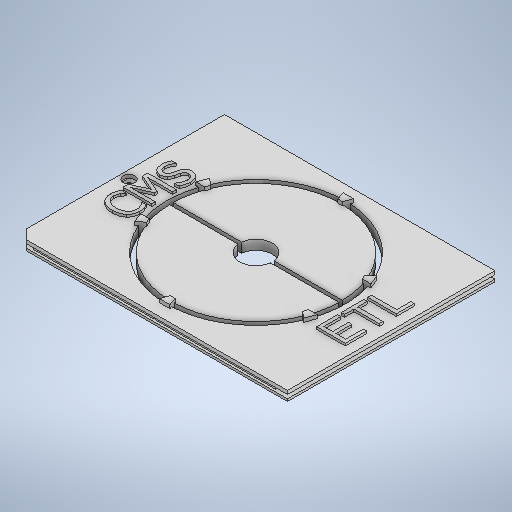
# Autodesk Inventor part: Tamale Souvenir
Saved by Autodesk Inventor 2025 (Build 290162000, 162)
## iProperties
Created: 2025-02-25
Part Number: Tamale Souvenir
Material: Generic
Document SubType Name: Modeling
Designer: Caleb Fangmeier
Density: 1 g/cm^3
Appearance: Default
Author: Caleb Fangmeier
Autodesk Inventor part; units mm, degrees
ref_plane "YZ Plane" through (0, 0, 0) normal (1, 0, 0) x (0, 1, 0)
ref_plane "XZ Plane" through (0, 0, 0) normal (0, 1, 0) x (-1, 0, 0)
ref_plane "XY Plane" through (0, 0, 0) normal (0, 0, 1) x (1, 0, 0)
sketch "Sketch1" plane through (0, 0, 0) normal (0, 1, 0) x (-1, 0, 0)
  line L0 (-28.75, -22.05) -> (28.75, -22.05)
  line L1 (28.75, -22.05) -> (28.75, 22.05)
  line L2 (28.75, 22.05) -> (-28.75, 22.05)
  line L3 (-28.75, 22.05) -> (-28.75, -22.05)
  line L4 (-28.75, -22.05) -> (28.75, 22.05) construction
  line L5 (28.75, -22.05) -> (-28.75, 22.05) construction
  point P0 (0, 0)
  dimension "d0" = 44.1
  dimension "d1" = 57.5
  constraints: 12 end point, 2 midpoint, 2 parallel, 1 horizontal, 1 perpendicular
  measures "d0" distance of L0.end L1.end
  measures "d1" distance of L1.end L2.end
extrude "Extrusion1" add sketch "Sketch1" along normal blind 0.5
sketch "Sketch2" plane through (0, 0.5, 0) normal (0, 1, 0) x (1, 0, 0)
  line L0 (-28.75, 22.05) -> (-28.75, -22.05) projected
  line L1 (-28.75, -22.05) -> (28.75, -22.05) projected
  line L2 (-28.75, -20.05) -> (-26.75, -22.05)
  point P0 (0, 0)
  dimension "d4" = 45
  dimension "d5" = 2
  constraints: 2 end point, 2 point on line
  measures "d4" angle of L2 L0
  measures "d5" distance of L2.start L0.end
extrude "Extrusion2" cut sketch "Sketch2" against normal through all
sketch "Sketch3" plane through (0, 0.5, 0) normal (0, 1, 0) x (1, 0, 0)
  line L0 (25.75, 21.55) -> (-25.75, 21.55)
  line L1 (-25.75, 21.55) -> (-25.75, -21.55)
  line L2 (-25.75, -21.55) -> (25.75, -21.55)
  line L3 (25.75, -21.55) -> (25.75, 21.55)
  line L4 (25.75, 21.55) -> (-25.75, -21.55) construction
  line L5 (-25.75, 21.55) -> (25.75, -21.55) construction
  line L6 (-26.75, -22.05) -> (28.75, -22.05) projected
  line L7 (-28.75, 22.05) -> (-28.75, -20.05) projected
  point P0 (0, 0)
  dimension "d8" = 0.5
  dimension "d9" = 3
  constraints: 12 end point, 2 midpoint, 2 parallel, 1 horizontal, 1 perpendicular
  measures "d8" distance between parallel lines of L6 L2
  measures "d9" distance between parallel lines of L7 L1
extrude "Extrusion3" add sketch "Sketch3" along normal blind 0.8
sketch "Sketch4" plane through (0, 1.3, 0) normal (0, 1, 0) x (1, 0, 0)
  line L0 (-25.75, 21.55) -> (-25.75, -21.55) projected
  line L1 (25.75, 0.25) -> (-25.75, 0.25)
  line L2 (-25.75, 0.25) -> (-25.75, -0.25)
  line L3 (-25.75, -0.25) -> (25.75, -0.25)
  line L4 (25.75, -0.25) -> (25.75, 0.25)
  line L5 (25.75, 0.25) -> (-25.75, -0.25) construction
  line L6 (-25.75, 0.25) -> (25.75, -0.25) construction
  line L7 (25.75, 21.55) -> (-25.75, 21.55) projected
  line L8 (0.25, -21.55) -> (-0.25, -21.55)
  line L9 (-0.25, -21.55) -> (-0.25, 21.55)
  line L10 (-0.25, 21.55) -> (0.25, 21.55)
  line L11 (0.25, 21.55) -> (0.25, -21.55)
  line L12 (0.25, -21.55) -> (-0.25, 21.55) construction
  line L13 (-0.25, -21.55) -> (0.25, 21.55) construction
  point P0 (0, 0)
  point P1 (0.25, -0.25)
  point P2 (0.25, 0.25)
  point P3 (-0.25, 0.25)
  point P4 (-0.25, -0.25)
  dimension "d12" = 0.5
  dimension "d13" = 0.5
  constraints: 24 end point, 4 midpoint, 4 parallel, 2 horizontal, 2 perpendicular, 2 point on line
  measures "d12" distance between parallel lines of L9 L11
  measures "d13" distance between parallel lines of L3 L1
extrude "Extrusion4" cut sketch "Sketch4" against normal up to surface (0.8 mm away) contours L1 L9 L3 L0 | L7 L11 L1 L9 | L1 L11 L3 L9 | L3 L11 L8 L9 | L1 L4 L3 L11
sketch "Sketch5" plane through (0, 1.3, 0) normal (0, 1, 0) x (1, 0, 0)
  line L0 (28.75, 22.05) -> (-28.75, 22.05)
  line L1 (-28.75, 22.05) -> (-28.75, -22.05)
  line L2 (-28.75, -22.05) -> (28.75, -22.05)
  line L3 (28.75, -22.05) -> (28.75, 22.05)
  line L4 (28.75, 22.05) -> (-28.75, -22.05) construction
  line L5 (-28.75, 22.05) -> (28.75, -22.05) construction
  point P0 (0, 0)
  constraints: 12 end point, 2 midpoint, 2 parallel, 1 coincident, 1 horizontal, 1 perpendicular
extrude "Extrusion5" add sketch "Sketch5" along normal blind 0.75
sketch "Sketch6" plane through (0, 2.05, 0) normal (0, 1, 0) x (1, 0, 0)
  line L0 (-28.75, 22.05) -> (-28.75, -22.05) projected
  line L1 (-28.75, -22.05) -> (28.75, -22.05) projected
  line L2 (-26.75, -22.05) -> (-28.75, -20.05) projected
  line L3 (-28.75, -20.05) -> (-26.75, -22.05)
  point P0 (0, 0)
  constraints: 2 end point, 1 collinear
extrude "Extrusion6" cut sketch "Sketch6" against normal through all
sketch "Sketch7" plane through (0, 2.05, 0) normal (0, 1, 0) x (1, 0, 0)
  circle A0 centre (0, 0) radius 19
  circle A1 centre (0, 0) radius 20
  dimension "d20" = 38
  dimension "d21" = 40
  constraints: 2 centre point, 2 coincident
  measures "d20" diameter of A0
  measures "d21" diameter of A1
extrude "Extrusion7" add sketch "Sketch7" against normal up to surface (2.05 mm away)
extrude "Extrusion8" cut sketch "Sketch7" against normal through all contours A0
sketch "Sketch8" plane through (0, 2.05, 0) normal (0, 1, 0) x (1, 0, 0)
  circle A0 centre (0, 0) radius 18
  circle A1 centre (0, 0) radius 19 projected
  dimension "d26" = 1
  constraints: 1 centre point, 1 coincident
  measures "d26" radial gap between concentric circles of A1 A0
extrude "Extrusion9" add sketch "Sketch8" against normal up to surface (2.05 mm away) contours A0
sketch "Sketch9" plane through (0, 2.05, 0) normal (0, 1, 0) x (1, 0, 0)
  line L0 (18.25, 0.375) -> (-18.25, 0.375)
  line L1 (-18.25, 0.375) -> (-18.25, -0.375)
  line L2 (-18.25, -0.375) -> (18.25, -0.375)
  line L3 (18.25, -0.375) -> (18.25, 0.375)
  line L4 (18.25, 0.375) -> (-18.25, -0.375) construction
  line L5 (-18.25, 0.375) -> (18.25, -0.375) construction
  point P0 (0, 0)
  dimension "d29" = 0.75
  dimension "d30" = 36.5
  constraints: 12 end point, 2 midpoint, 2 parallel, 1 horizontal, 1 perpendicular
  measures "d29" distance of L0.end L1.end
  measures "d30" distance of L0.start L0.end
extrude "Extrusion10" cut sketch "Sketch9" against normal blind 10
sketch "Sketch10" plane through (0, 2.05, 0) normal (0, 1, 0) x (1, 0, 0)
  line L0 (-16.4621, -6.804) -> (-16.8041, -5.8643)
  line L1 (-16.8041, -5.8643) -> (-18.6315, -5.8643)
  line L2 (-18.6315, -5.8643) -> (-17.8619, -7.9786)
  line L3 (-17.8619, -7.9786) -> (-16.4621, -6.804)
  line L4 (17.9961, -0.375) -> (-17.9961, -0.375) projected
  circle A0 centre (0, 0) radius 19 projected
  line L5 (0.608, -17.8024) -> (-0.392, -17.7937)
  line L6 (-0.392, -17.7937) -> (-1.032, -19.5053)
  line L7 (-1.032, -19.5053) -> (1.218, -19.525)
  line L8 (1.218, -19.525) -> (0.608, -17.8024)
  line L9 (16.8879, -5.6651) -> (16.5296, -6.5986)
  line L10 (16.5296, -6.5986) -> (17.9087, -7.7975)
  line L11 (17.9087, -7.7975) -> (18.715, -5.697)
  line L12 (18.715, -5.697) -> (16.8879, -5.6651)
  line L13 (-18.266, 0) -> (18.3496, 0)
  line L14 (-16.4621, 6.804) -> (-16.8041, 5.8643)
  line L15 (-16.8041, 5.8643) -> (-18.6315, 5.8643)
  line L16 (-18.6315, 5.8643) -> (-17.8619, 7.9786)
  line L17 (-17.8619, 7.9786) -> (-16.4621, 6.804)
  line L18 (0.608, 17.8024) -> (-0.392, 17.7937)
  line L19 (-0.392, 17.7937) -> (-1.032, 19.5053)
  line L20 (-1.032, 19.5053) -> (1.218, 19.525)
  line L21 (1.218, 19.525) -> (0.608, 17.8024)
  line L22 (16.8879, 5.6651) -> (16.5296, 6.5986)
  line L23 (16.5296, 6.5986) -> (17.9087, 7.7975)
  line L24 (17.9087, 7.7975) -> (18.715, 5.697)
  line L25 (18.715, 5.697) -> (16.8879, 5.6651)
  dimension "d33" = 1
  dimension "d34" = 2.25
  dimension "d35" = 110
  dimension "d36" = 110
  dimension "d37" = 110
  dimension "d41" = 139
  constraints: 50 end point, 12 symmetric about line, 1 horizontal, 1 parallel, 17 other
  measures "d33" distance of L0.start L0.end
  measures "d34" distance of L1.end L2.end
  measures "d35" angle of L0 L1
  measures "d36" angle of L3 L0
  measures "d37" angle of L4 L2
extrude "Extrusion11" add sketch "Sketch10" along normal blind 0.75 and the other way blind 2.05 contours L3 A0 L1 L0 | L3 L2 L1 A0 | L6 L5 L8 A0 | A0 L8 L7 L6 | L15 L16 L17 A0 | A0 L17 L14 L15 | L10 L9 L12 A0 | A0 L12 L11 L10 | L19 L20 L21 A0 | A0 L21 L18 L19 | L23 L24 L25 A0 | A0 L25 L22 L23
sketch "Sketch11" plane through (0, 2.05, 0) normal (0, 1, 0) x (1, 0, 0)
  circle A0 centre (0, 0) radius 3.4726
  constraints: 1 centre point, 1 coincident
extrude "Extrusion12" cut sketch "Sketch11" against normal through all
sketch "Sketch12" plane through (0, 2.05, 0) normal (0, 1, 0) x (1, 0, 0)
  line L0 (-28.75, 22.05) -> (-28.75, -20.05) projected
  line L1 (20.6121, -8.4043) -> (20.6121, 11.3007) construction
  line L2 (20.6121, 11.3007) -> (27.7105, 11.3007) construction
  line L3 (27.7105, 11.3007) -> (27.7105, -8.4043) construction
  line L4 (27.7105, -8.4043) -> (20.6121, -8.4043) construction
  line L5 (-25.7514, -8.2683) -> (-25.7514, -0.1864) construction
  line L6 (-25.7514, -0.1864) -> (-22.5947, -0.1864) construction
  line L7 (-22.5947, -0.1864) -> (-22.5947, -8.2683) construction
  line L8 (-22.5947, -8.2683) -> (-25.7514, -8.2683) construction
  spline S0 degree 2 poles (-19.4339, -5.2678) (-19.4339, -5.861) (-19.8343, -6.8644) (-20.2347, -7.2302) knots 0 0 0 1 2 2 2
  spline S1 degree 2 poles (-20.2347, -7.2302) (-20.6302, -7.596) (-21.8166, -7.9964) (-22.5877, -7.9964) knots 0 0 0 1 2 2 2
  spline S2 degree 2 poles (-22.5877, -7.9964) (-23.3539, -7.9964) (-24.4909, -7.6059) (-24.911, -7.2352) knots 0 0 0 1 2 2 2
  spline S3 degree 2 poles (-24.911, -7.2352) (-25.3213, -6.8694) (-25.7514, -5.8708) (-25.7514, -5.2529) knots 0 0 0 1 2 2 2
  spline S4 degree 2 poles (-25.7514, -5.2529) (-25.7514, -4.9464) (-25.6624, -4.4076) (-25.5932, -4.1802) knots 0 0 0 1 2 2 2
  spline S5 degree 2 poles (-25.5932, -4.1802) (-25.529, -3.9825) (-25.3461, -3.5722) (-25.2373, -3.3695) knots 0 0 0 1 2 2 2
  line L9 (-25.2373, -3.3695) -> (-24.2585, -3.3695)
  line L10 (-24.2585, -3.3695) -> (-24.2585, -3.4338)
  spline S6 degree 2 poles (-24.2585, -3.4338) (-24.3574, -3.5426) (-24.6342, -3.8787) (-24.7677, -4.1209) knots 0 0 0 1 2 2 2
  spline S7 degree 2 poles (-24.7677, -4.1209) (-24.8962, -4.3533) (-25.0593, -4.902) (-25.0593, -5.2579) knots 0 0 0 1 2 2 2
  spline S8 degree 2 poles (-25.0593, -5.2579) (-25.0593, -5.6484) (-24.738, -6.3454) (-24.4315, -6.6074) knots 0 0 0 1 2 2 2
  spline S9 degree 2 poles (-24.4315, -6.6074) (-24.1201, -6.8644) (-23.176, -7.1511) (-22.5877, -7.1511) knots 0 0 0 1 2 2 2
  spline S10 degree 2 poles (-22.5877, -7.1511) (-21.9599, -7.1511) (-21.0553, -6.8496) (-20.7439, -6.5876) knots 0 0 0 1 2 2 2
  spline S11 degree 2 poles (-20.7439, -6.5876) (-20.4423, -6.3306) (-20.1358, -5.6435) (-20.1358, -5.2579) knots 0 0 0 1 2 2 2
  spline S12 degree 2 poles (-20.1358, -5.2579) (-20.1358, -4.9069) (-20.3089, -4.3088) (-20.4374, -4.0764) knots 0 0 0 1 2 2 2
  spline S13 degree 2 poles (-20.4374, -4.0764) (-20.5659, -3.854) (-20.8328, -3.5228) (-20.9268, -3.4289) knots 0 0 0 1 2 2 2
  line L11 (-20.9268, -3.4289) -> (-20.9268, -3.3695)
  line L12 (-20.9268, -3.3695) -> (-19.9579, -3.3695)
  spline S14 degree 2 poles (-19.9579, -3.3695) (-19.864, -3.5722) (-19.6909, -3.9281) (-19.6119, -4.1802) knots 0 0 0 1 2 2 2
  spline S15 degree 2 poles (-19.6119, -4.1802) (-19.5229, -4.4472) (-19.4339, -4.902) (-19.4339, -5.2678) knots 0 0 0 1 2 2 2
  line L13 (-19.5427, 2.6168) -> (-19.5427, 1.8061)
  line L14 (-19.5427, 1.8061) -> (-24.7974, 1.8061)
  line L15 (-24.7974, 1.8061) -> (-21.2234, 0.2143)
  line L16 (-21.2234, 0.2143) -> (-21.2234, -0.28)
  line L17 (-21.2234, -0.28) -> (-24.7974, -1.8569)
  line L18 (-24.7974, -1.8569) -> (-19.5427, -1.8569)
  line L19 (-19.5427, -1.8569) -> (-19.5427, -2.6132)
  line L20 (-19.5427, -2.6132) -> (-25.6427, -2.6132)
  line L21 (-25.6427, -2.6132) -> (-25.6427, -1.5059)
  line L22 (-25.6427, -1.5059) -> (-22.2466, 0.0166)
  line L23 (-22.2466, 0.0166) -> (-25.6427, 1.4897)
  line L24 (-25.6427, 1.4897) -> (-25.6427, 2.6168)
  line L25 (-25.6427, 2.6168) -> (-19.5427, 2.6168)
  spline S16 degree 2 poles (-19.4339, 5.5531) (-19.4339, 4.8907) (-19.7107, 3.9613) (-19.9085, 3.551) knots 0 0 0 1 2 2 2
  line L26 (-19.9085, 3.551) -> (-20.9268, 3.551)
  line L27 (-20.9268, 3.551) -> (-20.9268, 3.6104)
  spline S17 degree 2 poles (-20.9268, 3.6104) (-20.5511, 4.0108) (-20.1358, 5.0241) (-20.1358, 5.4937) knots 0 0 0 1 2 2 2
  spline S18 degree 2 poles (-20.1358, 5.4937) (-20.1358, 6.166) (-20.6944, 6.8531) (-21.1542, 6.8531) knots 0 0 0 1 2 2 2
  spline S19 degree 2 poles (-21.1542, 6.8531) (-21.52, 6.8531) (-21.9747, 6.4923) (-22.0884, 6.1018) knots 0 0 0 1 2 2 2
  spline S20 degree 2 poles (-22.0884, 6.1018) (-22.1675, 5.82) (-22.2763, 5.3504) (-22.3653, 4.9994) knots 0 0 0 1 2 2 2
  spline S21 degree 2 poles (-22.3653, 4.9994) (-22.4493, 4.683) (-22.7014, 4.1838) (-22.9041, 3.991) knots 0 0 0 1 2 2 2
  spline S22 degree 2 poles (-22.9041, 3.991) (-23.1068, 3.8031) (-23.6505, 3.5955) (-24.0064, 3.5955) knots 0 0 0 1 2 2 2
  spline S23 degree 2 poles (-24.0064, 3.5955) (-24.7479, 3.5955) (-25.7514, 4.7523) (-25.7514, 5.647) knots 0 0 0 1 2 2 2
  spline S24 degree 2 poles (-25.7514, 5.647) (-25.7514, 6.1611) (-25.5487, 7.0706) (-25.3559, 7.4612) knots 0 0 0 1 2 2 2
  line L28 (-25.3559, 7.4612) -> (-24.3871, 7.4612)
  line L29 (-24.3871, 7.4612) -> (-24.3871, 7.4018)
  spline S25 degree 2 poles (-24.3871, 7.4018) (-24.654, 7.1102) (-25.0495, 6.2006) (-25.0495, 5.7014) knots 0 0 0 1 2 2 2
  spline S26 degree 2 poles (-25.0495, 5.7014) (-25.0495, 5.1378) (-24.5205, 4.4408) (-24.0905, 4.4408) knots 0 0 0 1 2 2 2
  spline S27 degree 2 poles (-24.0905, 4.4408) (-23.7049, 4.4408) (-23.2452, 4.8511) (-23.1414, 5.2367) knots 0 0 0 1 2 2 2
  spline S28 degree 2 poles (-23.1414, 5.2367) (-23.0721, 5.4937) (-22.8942, 6.2402) (-22.82, 6.4873) knots 0 0 0 1 2 2 2
  spline S29 degree 2 poles (-22.82, 6.4873) (-22.6273, 7.1151) (-21.8512, 7.6984) (-21.2827, 7.6984) knots 0 0 0 1 2 2 2
  spline S30 degree 2 poles (-21.2827, 7.6984) (-20.9218, 7.6984) (-20.2298, 7.4068) (-19.9875, 7.1448) knots 0 0 0 1 2 2 2
  spline S31 degree 2 poles (-19.9875, 7.1448) (-19.7206, 6.8531) (-19.4339, 6.1117) (-19.4339, 5.5531) knots 0 0 0 1 2 2 2
  line L30 (26.7121, -7.7302) -> (20.6121, -7.7302)
  line L31 (20.6121, -7.7302) -> (20.6121, -3.3132)
  line L32 (20.6121, -3.3132) -> (21.3328, -3.3132)
  line L33 (21.3328, -3.3132) -> (21.3328, -6.9212)
  line L34 (21.3328, -6.9212) -> (23.1972, -6.9212)
  line L35 (23.1972, -6.9212) -> (23.1972, -3.5411)
  line L36 (23.1972, -3.5411) -> (23.9179, -3.5411)
  line L37 (23.9179, -3.5411) -> (23.9179, -6.9212)
  line L38 (23.9179, -6.9212) -> (25.9915, -6.9212)
  line L39 (25.9915, -6.9212) -> (25.9915, -3.1738)
  line L40 (25.9915, -3.1738) -> (26.7121, -3.1738)
  line L41 (26.7121, -3.1738) -> (26.7121, -7.7302)
  line L42 (26.7121, -0.5097) -> (21.3328, -0.5097)
  line L43 (21.3328, -0.5097) -> (21.3328, -2.5182)
  line L44 (21.3328, -2.5182) -> (20.6121, -2.5182)
  line L45 (20.6121, -2.5182) -> (20.6121, 2.3172)
  line L46 (20.6121, 2.3172) -> (21.3328, 2.3172)
  line L47 (21.3328, 2.3172) -> (21.3328, 0.2993)
  line L48 (21.3328, 0.2993) -> (26.7121, 0.2993)
  line L49 (26.7121, 0.2993) -> (26.7121, -0.5097)
  line L50 (26.7121, 3.1122) -> (20.6121, 3.1122)
  line L51 (20.6121, 3.1122) -> (20.6121, 3.9212)
  line L52 (20.6121, 3.9212) -> (25.9915, 3.9212)
  line L53 (25.9915, 3.9212) -> (25.9915, 6.9247)
  line L54 (25.9915, 6.9247) -> (26.7121, 6.9247)
  line L55 (26.7121, 6.9247) -> (26.7121, 3.1122)
  point P0 (0, 0)
  constraints: 2 parallel, 4 other
emboss "Emboss1" sketch "Sketch12" operation add depth 0.5 direction (0, -1, 0)
sketch "Sketch13" plane through (0, 2.05, 0) normal (0, 1, 0) x (1, 0, 0)
  circle A0 centre (-26.9813, 0) radius 1.25
  point P0 (0, 0)
  dimension "d52" = 2.5
  constraints: 1 centre point
  measures "d52" diameter of A0
extrude "Extrusion13" cut sketch "Sketch13" against normal through all
equation "\"d36\" = d35"
body "Solid1"
